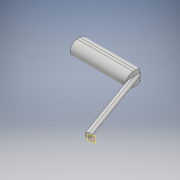
# Autodesk Inventor part: Haut du manche
Saved by Autodesk Inventor 2018.1 (Build 221171000, 171)
## iProperties
Created: 2019-11-15
Part Number: Haut du manche
Material: Générique
Document SubType Name: Modeling
Designer: ageib2
Density: 1 g/cm^3
Appearance: Par défaut
Author: ageib2
Autodesk Inventor part; units mm, degrees
ref_plane "YZ Plane" through (0, 0, 0) normal (1, 0, 0) x (0, 1, 0)
ref_plane "XZ Plane" through (0, 0, 0) normal (0, 1, 0) x (-1, 0, 0)
ref_plane "XY Plane" through (0, 0, 0) normal (0, 0, 1) x (1, 0, 0)
sketch "Esquisse1" plane through (0, 0, 0) normal (0, 0, 1) x (1, 0, 0)
  line L0 (-100, 30) -> (100, 30)
  line L1 (100, 30) -> (100, -30)
  line L2 (100, -30) -> (-100, -30)
  line L3 (-100, -30) -> (-100, 30)
  point P0 (0, 0)
  dimension "d0" = 200
  dimension "d1" = 60
  dimension "d2" = 100
  dimension "d3" = 30
  constraints: 8 end point, 2 parallel, 1 horizontal, 1 perpendicular
  measures "d0" distance of L1.end L2.end
  measures "d1" distance of L0.end L1.end
  measures "d2" distance from line of L1 point (0, 0)
  measures "d3" distance from line of point (0, 0) L0
extrude "Extrusion1" add sketch "Esquisse1" along normal blind 50
fillet "Congé1" radius 25 4 edges at (0, 30, 50) (0, 30, 0) (0, -30, 50) (0, -30, 0)
ref_plane "Plan de construction6" through (201.1224, -254.4412, 16.7193) normal (0.3420201, -0.9396926, 0) x (0.9396926, 0.3420201, 0)
sketch "Esquisse5" plane through (201.1224, -254.4412, 16.7193) normal (0.3420201, -0.9396926, 0) x (0.9396926, 0.3420201, 0)
  line L0 (-7.928, 15.9556) -> (-15.928, 15.9556)
  line L1 (-7.928, -0.0444) -> (-15.928, -0.0444)
  line L2 (-15.928, -0.0444) -> (-15.928, 15.9556)
  arc A0 (-7.428, -0.0444) -> (0.072, 7.9556) centre (-8.3118, 8.2999) ccw
  arc A1 (0.072, 7.9556) -> (-7.428, 15.9556) centre (-7.1293, 8.72) ccw
  line L3 (-15.928, -0.0444) -> (-7.428, -0.0444)
  line L4 (-15.928, 15.9556) -> (-7.428, 15.9556)
  point P0 (-101.9693, -16.7193)
  constraints: 10 end point, 4 point on circle, 2 centre point
extrude "Extrusion3" add sketch "Esquisse5" against normal through all
sketch "Esquisse6" plane through (0, 0, 50) normal (0, 0, 1) x (1, 0, 0)
  line L0 (100, 30) -> (100, 5) projected
  line L1 (100, 30) -> (100, 23.601)
  line L2 (100, 23.601) -> (45.7922, 30)
  line L3 (100, 30) -> (-100, 30) projected
  point P0 (0, 0)
  dimension "d20" = 6.399
  constraints: 4 end point, 2 point on line
  measures "d20" distance of L0.start L1.end
extrude "Extrusion4" cut sketch "Esquisse6" against normal through all
fillet "Congé2" radius 5 2 edges at (100, 23.601, 33.9536) (100, 23.601, 16.4857)
